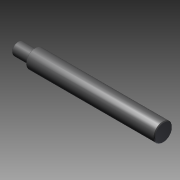
# Autodesk Inventor part: SSFCU12-85-F12-P8
Saved by Autodesk Inventor 2011 SP1 (Build 150282100, 282)
## iProperties
Created: 2016-11-09
Part Number: SSFCU12-85-F12-P8
Catalog Web Link: www.cadenas.de
Description: SFAC, SSFAC, PSFAC, PSSFAC, RSFAC, SFCU, SSFCU, PSFCU, PSSFCU, PSCGC, PSSCGC-Shafts - One End Stepped
Vendor: MISUMI
Document SubType Name: Modeling
Designer: psAdmin
Manufacturer: MISUMI
Mass: 10.1902 g
Surface Area: 36.8585 cm^2
Volume: 10.1902 cm^3
Density: 1 g/cm^3
Category: PARTsolutions
Company: MISUMI
Title: SSFCU12-85-F12-P8
Author: Cadenas PARTsolutions
Comments: Shafts - One End Stepped
PSOL_IDENT_0: {$CADENAS_DATA\23d-libs\misumi\metric\01_linear_shafts\pscgc.prj},334 {VTYP=3D},{NB=SSFCU12-85-F12-P
PSOL_IDENT_1: 8},{LINA=SSFCU12-85-F12-P8},{NN=SFAC, SSFAC, PSFAC, PSSFAC, RSFAC, SFCU, SSFCU, PSFCU, PSSFCU, PSCGC
PSOL_IDENT_2: , PSSCGC},{DATE=17.06.2016 05:45:06},{GEOMDATE=10.12.2015 06:08:53},{VERSION=},{LINEID=70},{LINESUBI
PSOL_IDENT_3: D=-1},{WBVAR=DTS,MAT,ST,ALT1,L,F,P,ALT4,FC,WFC,A,E,ALT5,RC,WRC,YALT5,ALT7,WKC,C,KC,G,ALT22,LFC,AALT2
PSOL_IDENT_4: 2}  {NB=SSFCU12-85-F12-P8},{LINA=SSFCU12-85-F12-P8},{KT=DUMMY},{PN=SSFCU12-85-F12-P8},{TYPE=SSFCU},{
PSOL_IDENT_5: DTS=h5},{DTSALG= 'g6','g6','h5','h5','f8','f8' },{MAT=SUS440C},{MATALG= 'SUJ2','SUJ2','SUS440C','SUS
PSOL_IDENT_6: 440C Equivalent' },{ST=-},{STALG= '-','-','HCP5','Hard Chrome Plating - Plating Hardness: HV750~ Pla
PSOL_IDENT_7: ting Thickness: 5 micron or More' },{D=12},{ALT1=},{ALT1ALG= '','w/o LKC (L Dimension Tolerance Chan
PSOL_IDENT_8: ge)','LKC','with LKC (L Dimension Tolerance Change)' },{ALT1PN=},{L=85.0},{LALG=[25:1198/1]},{LMIN=2
PSOL_IDENT_9: 5},{LMAX=1198},{F=12},{FALG=[2:40/1]},{FMIN=2},{FMAX=40},{P=8},{PALG=[6:10/1]},{PMIN=6},{PMIN1=6},{P
PSOL_IDENT_10: MIN2=3},{PMAX=10},{Y=1200},{R=0.3},{CIFR=0},{CIFRCUT=0},{LSC=0.5},{RSC=0.5},{CP=1.25},{CPALG=8},{CPP
PSOL_IDENT_11: ITCH=1.25},{CIFLSC=0},{ALT4=},{ALT4ALG= '','w/o Set Screw Flat','FC','with FC (Set Screw Flat at One
PSOL_IDENT_12: Location)','WFC','with WFC (Set Screw Flats at Two Locations)' },{ALT4PN=},{FC=0},{FCALG=[0]},{FCMA
PSOL_IDENT_13: X=60},{WFC=0},{WFCALG=[0]},{WFCMAX=41},{A=0},{AALG=[0]},{AMAX=0},{E=0},{EALG=[0]},{EMAX=0},{HHALT4=0
PSOL_IDENT_14: },{FC3D=0},{CIFE=0},{CIFA=0},{ALT5=},{ALT5ALG= '','w/o 90-deg. Set Screw Flat','RC','with RC (90-deg
PSOL_IDENT_15: . Set Screw Flat at One Location)','WRC','with WRC (90-deg. Set Screw Flats at Two Locations)' },{AL
PSOL_IDENT_16: T5PN=},{RC=0},{RCALG=[0]},{RCMIN=2},{RCMAX=85},{WRC=0},{WRCALG=[0]},{WRCMIN=2},{WRCMAX=81},{RC3D=0},
PSOL_IDENT_17: {YALT5=0},{YALT5ALG=[0]},{YALT5MIN=2},{YALT5MAX=83},{BB1=0},{BB1ALG=6},{HHALT5=0.0},{CIFRC=0},{CIFY=
PSOL_IDENT_18: 0},{ALT7=},{ALT7ALG= '','w/o Add Keyway' , 'KC','with KC (Add Keyway at One Location)','WKC','with W
PSOL_IDENT_19: KC (Adds Keyways at Two Locations)' },{ALT7PN=},{WKC=0},{WKCALG=[0]},{WKCMAX=83},{C=0},{CALG=[0]},{C
PSOL_IDENT_20: MIN=0},{CMAX=30},{KC=0},{KCALG=[0]},{KCMAX1=83},{KCMAX2=85},{KCMAX3=83},{G=0},{GALG=[0]},{GMIN=0},{G
PSOL_IDENT_21: MAX1=30},{GMAX2=30},{GMAX3=30},{BB=0},{TT=0.0},{CIFKC=0},{CIFWKC=1},{ALT22=},{ALT22ALG= '','w/o LFC
PSOL_IDENT_22: (Left Side Set Screw Flat at Step)','LFC','with LFC (Left Side Set Screw Flat at Step)' },{ALT22PN=}
PSOL_IDENT_23: ,{LFC=0},{LFCALG=[0]},{LFCMIN=3},{LFCMAX=12},{AALT22=0},{AALT22ALG=[0]},{AALT22MIN=2},{AALT22MAX=12}
PSOL_IDENT_24: ,{H=0},{ERRORPN=},{ERRORALT45=OK},{ERRORALT47=OK},{ERRORALT57=OK},{ERRORALT722=OK}
NN: SFAC, SSFAC, PSFAC, PSSFAC, RSFAC, SFCU, SSFCU, PSFCU, PSSFCU, PSCGC, PSSCGC
NT: Shafts - One End Stepped
NB: SSFCU12-85-F12-P8
NBSYN: $PN.
LINA: SSFCU12-85-F12-P8
PN: SSFCU12-85-F12-P8
DTS: h5
MAT: SUS440C Equivalent
ST: -
D: 12
ALT1: w/o LKC (L Dimension Tolerance Change)
L: 85.0
F: 12
P: 8
Y: 1200
R: 0.3
LSC: 0.5
RSC: 0.5
ALT4: w/o Set Screw Flat
FC: 0
WFC: 0
A: 0
E: 0
HHALT4: 0
ALT5: w/o 90-deg. Set Screw Flat
RC: 0
WRC: 0
YALT5: 0
BB1: 0
HHALT5: 0.0
ALT7: w/o Add Keyway
WKC: 0
C: 0
KC: 0
G: 0
BB: 0
TT: 0.0
ALT22: w/o LFC (Left Side Set Screw Flat at Step)
LFC: 0
AALT22: 0
H: 0
SUPPLIER: MISUMI
ARTICLENO: SSFCU12-85-F12-P8
BOMINFO: SSFCU12-85-F12-P8
CREATOR: CADENAS GmbH
Autodesk Inventor part; units mm, degrees
ref_plane "YZ Plane" through (0, 0, 0) normal (1, 0, 0) x (0, 1, 0)
ref_plane "XZ Plane" through (0, 0, 0) normal (0, 1, 0) x (-1, 0, 0)
ref_plane "XY Plane" through (0, 0, 0) normal (0, 0, 1) x (1, 0, 0)
sketch "Sketch_1" plane through (0, 0, 0) normal (0, 0, 1) x (1, 0, 0)
  line L0 (85, 0) -> (-12, 0)
  line L1 (-12, 0) -> (-12, 2.75)
  line L2 (-12, 2.75) -> (-10.75, 4)
  line L3 (-10.75, 4) -> (-0.3, 4)
  arc A0 (-0.3, 4) -> (0, 4.3) centre (-0.3, 4.3) ccw
  line L4 (0, 4.3) -> (0, 5.5)
  line L5 (0, 5.5) -> (0.5, 6)
  line L6 (0.5, 6) -> (84.5, 6)
  line L7 (84.5, 6) -> (85, 5.5)
  line L8 (85, 5.5) -> (85, 0)
  line L9 (85, 0) -> (-12, 0)
  constraints: 20 end point, 2 point on circle, 1 centre point
revolve "Revolution1" add sketch "Sketch_1" angle 360 about axis through (85, 0, 0) along (1, 0, 0)
body "Solid1"
